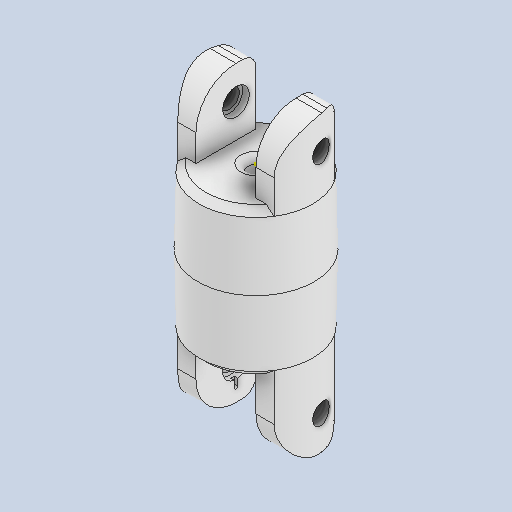
# Autodesk Inventor part: Index_1
Saved by Autodesk Inventor 2022 (Build 260153000, 153)
## iProperties
Created: 2023-01-15
Part Number: Index_1
Material: ABS Plastic
Document SubType Name: Modeling
Designer: 48735
Density: 1.06 g/cm^3
Appearance: Smooth - White
Author: 48735
Autodesk Inventor part; units mm, degrees
ref_plane "YZ Plane" through (0, 0, 0) normal (1, 0, 0) x (0, 1, 0)
ref_plane "XZ Plane" through (0, 0, 0) normal (0, 1, 0) x (-1, 0, 0)
ref_plane "XY Plane" through (0, 0, 0) normal (0, 0, 1) x (1, 0, 0)
sketch "Sketch1" plane through (0, 0, 0) normal (0, 1, 0) x (-1, 0, 0)
  line L0 (4.5, 0) -> (4.5, -4)
  line L1 (4.5, 0) -> (4.5, 4)
  line L2 (-4.5, 0) -> (-4.5, -4)
  line L3 (-4.5, 0) -> (-4.5, 4)
  circle A0 centre (0, 0) radius 8.5
  line L4 (4.5, 4) -> (4.5, 4.5)
  line L5 (-4.5, 4) -> (-4.5, 4.5)
  line L6 (-4.5, -4) -> (-4.5, -4.5)
  line L7 (-4.5, -4.5) -> (-7.2111, -4.5)
  line L8 (4.5, -4) -> (4.5, -4.5)
  line L9 (4.5, -4.5) -> (7.2111, -4.5)
  line L10 (4.5, 4) -> (4.5, 4.5)
  line L11 (4.5, 4.5) -> (7.2111, 4.5)
  line L12 (-4.5, 4) -> (-4.5, 4.5)
  line L13 (-4.5, 4.5) -> (-7.2111, 4.5)
  point P0 (7.5, 4)
  point P1 (7.5, -4)
  point P2 (-7.5, -4)
  point P3 (-7.5, 4)
  constraints: 28 end point, 3 point on line, 2 parallel, 2 perpendicular, 2 vertical, 1 coincident, 10 other
extrude "Extrusion1" add sketch "Sketch1" along normal blind 12 contours L1 L4 L11 A0 L9 L8 L0 | A0 L13 L5 L3 L2 L6 L7
sketch "Sketch2" plane through (0, 12, 0) normal (0, 1, 0) x (1, 0, 0)
  circle A0 centre (0, 0) radius 8.5
  circle A1 centre (0, 0) radius 1.25
  dimension "d11" = 17
  dimension "d12" = 2.5
  constraints: 2 centre point, 2 coincident
  measures "d11" diameter of A0
  measures "d12" diameter of A1
extrude "Extrusion2" add sketch "Sketch2" along normal blind 1
fillet "Fillet4" radius 6 2 edges at (-5.8556, 0, 4.5) (5.8556, 0, 4.5)
fillet "Fillet5" radius 2 2 edges at (5.8556, 0, -4.5) (-5.8556, 0, -4.5)
sketch "Sketch4" plane through (4.5, 12, -4.5) normal (-1, 0, 0) x (0, 0, 1)
  arc A0 (3, -12) -> (9, -6) centre (3, -6) ccw projected
  line L0 (3, -12) -> (3, -7)
  point P0 (4.5, -12)
  dimension "d30" = 5
  constraints: 2 end point, 1 vertical
  measures "d30" distance of L0.start L0.end
hole "Hole2" at (4.5, 5, -1.5) direction (1, 0, 0) diameter 3 depth 5 counterbore diameter 4 counterbore depth 1
sketch "Sketch5" plane through (-4.5, 12, 4.5) normal (1, 0, 0) x (0, 0, -1)
  line L0 (6, -12) -> (6, -7)
  point P0 (4.5, -12)
  dimension "d38" = 5
  constraints: 2 end point, 1 vertical
  measures "d38" distance of L0.start L0.end
hole "Hole3" at (-4.5, 5, -1.5) direction (-1, 0, 0) diameter 3 depth 5 counterbore diameter 4 counterbore depth 1
sketch "Sketch8" plane through (4.5, 12, -4.5) normal (-1, 0, 0) x (0, 0, 1)
  circle A0 centre (3, -7) radius 2 projected
  line L0 (3.25, -7) -> (3.25, -10)
  line L1 (2.75, -7) -> (2.75, -10)
  line L2 (3.25, -7) -> (2.75, -7)
  arc A1 (2.75, -10) -> (3.25, -10) centre (3, -10) ccw
  point P0 (4.5, -12)
  constraints: 6 end point, 2 point on circle, 1 centre point
extrude "Extrusion5" cut sketch "Sketch8" against normal blind 0.5 contours L1 L2 L0 A0 | A0 L0 A1 L1 picked at (2.9722, -7.6661)
sketch "Sketch9" plane through (5, 12, -4.5) normal (-1, 0, 0) x (0, 0, 1)
  arc A0 (2.75, -10) -> (3.25, -10) centre (3, -10) ccw projected
  circle A1 centre (3, -10) radius 0.25
  point P0 (4.5, -12)
  constraints: 1 centre point, 1 coincident
extrude "Extrusion6" cut sketch "Sketch9" against normal blind 0.5
sketch "Sketch10" plane through (-4.5, 12, 4.5) normal (1, 0, 0) x (0, 0, -1)
  circle A0 centre (6, -7) radius 2 projected
  line L0 (6.25, -7) -> (6.25, -10)
  line L1 (5.75, -7) -> (5.75, -10)
  line L2 (5.75, -7) -> (6.25, -7)
  arc A1 (5.75, -10) -> (6.25, -10) centre (6, -10) ccw
  point P0 (4.5, -12)
  constraints: 6 end point, 2 point on circle, 1 centre point
extrude "Extrusion7" cut sketch "Sketch10" against normal blind 0.5 contours L1 L2 L0 A0 | A0 L0 A1 L1 picked at (6.0278, -7.6661)
sketch "Sketch11" plane through (-5, 12, 4.5) normal (1, 0, 0) x (0, 0, -1)
  arc A0 (5.75, -10) -> (6.25, -10) centre (6, -10) ccw projected
  circle A1 centre (6, -10) radius 0.25
  point P0 (4.5, -12)
  constraints: 1 centre point, 1 coincident
extrude "Extrusion8" cut sketch "Sketch11" against normal blind 0.5
chamfer "Chamfer3" distance 1 angle 45 2 edges at (0, 12, 8.5) (0, 12, -8.5)
fillet "Fillet6" radius 1 1 edges at (-1.25, 12, 0)
sketch "Sketch12" plane through (0, 13, 0) normal (0, 1, 0) x (1, 0, 0)
  circle A0 centre (0, 0) radius 1.25
  circle A1 centre (0, 0) radius 8.7
  dimension "d79" = 17.4
  constraints: 2 centre point, 2 coincident
  measures "d79" diameter of A1
extrude "Extrusion9" add sketch "Sketch12" along normal blind 10
chamfer "Chamfer4" distance 10 distance2 0.2 1 edges at (-8.7, 13, 0) measured on face at (8.5873, 19.6667, 1.3956)
sketch "Sketch13" plane through (0, 23, 0) normal (0, 1, 0) x (1, 0, 0)
  circle A0 centre (0, 0) radius 1.25
  circle A1 centre (0, 0) radius 8.7
  dimension "d83" = 17.4
  constraints: 2 centre point, 2 coincident
  measures "d83" diameter of A1
extrude "Extrusion10" add sketch "Sketch13" along normal blind 10
chamfer "Chamfer5" distance 0.2 distance2 10 1 edges at (-8.7, 33, 0) measured on face at (6.1324, 33, 0.694)
sketch "Sketch14" plane through (0, 33, 0) normal (0, 1, 0) x (1, 0, 0)
  circle A0 centre (0, 0) radius 8.5
  circle A1 centre (0, 0) radius 1.25
  dimension "d91" = 17
  dimension "d90" = 2.5
  constraints: 2 centre point, 2 coincident
  measures "d91" diameter of A0
  measures "d90" diameter of A1
extrude "Extrusion11" add sketch "Sketch14" along normal blind 1
fillet "Fillet7" radius 1 1 edges at (-1.25, 34, 0)
sketch "Sketch15" plane through (0, 34, 0) normal (0, 1, 0) x (1, 0, 0)
  point P0 (0, 0)
sketch "Sketch16" plane through (0, 34, 0) normal (0, 1, 0) x (1, 0, 0)
  circle A0 centre (0, 0) radius 2.25 projected
  circle A1 centre (0, 0) radius 8.5
  circle A2 centre (0, 0) radius 1.25 projected
  line L0 (4.5, 0) -> (4.5, 4.5)
  line L1 (4.5, 4.5) -> (7.2111, 4.5)
  line L2 (4.5, -4.5) -> (4.5, 1.5) projected
  line L3 (4.5, 0) -> (4.5, -4.5)
  line L4 (7.2111, -4.5) -> (4.5, -4.5) projected
  line L5 (4.5, -4.5) -> (7.2111, -4.5)
  line L6 (-7.2111, 4.5) -> (-4.5, 4.5) projected
  line L7 (-4.5, 0) -> (-4.5, 4.5)
  line L8 (-4.5, 4.5) -> (-7.2111, 4.5)
  line L9 (-4.5, 0) -> (-4.5, -4.5)
  line L10 (-4.5, 1.5) -> (-4.5, -4.5) projected
  line L11 (-4.5, -4.5) -> (-7.2111, -4.5)
  point P0 (-7.2111, -4.5)
  point P1 (-7.2111, -4.5)
  constraints: 16 end point, 2 point on circle, 1 centre point, 1 coincident, 1 perpendicular, 1 vertical
extrude "Extrusion12" add sketch "Sketch16" along normal blind 10 contours A1 L4 L2 L0 L1 | L6 L7 L9 L11 A1
chamfer "Chamfer6" distance 1 angle 45 2 edges at (0, 34, 8.5) (0, 34, -8.5)
fillet "Fillet8" radius 6 2 edges at (-5.8556, 44, 4.5) (5.8556, 44, 4.5)
fillet "Fillet9" radius 2 2 edges at (5.8556, 44, -4.5) (-5.8556, 44, -4.5)
sketch "Sketch17" plane through (-4.5, 34, 4.5) normal (1, 0, 0) x (0, 0, -1)
  line L0 (6, 10) -> (7, 10) projected
  line L1 (6, 10) -> (6, 5)
  point P0 (4.5, -34)
  dimension "d106" = 5
  constraints: 2 end point, 1 vertical
  measures "d106" distance of L0.start L1.end
hole "Hole4" at (-4.5, 39, -1.5) direction (-1, 0, 0) diameter 3 depth 5 counterbore diameter 4 counterbore depth 1
sketch "Sketch18" plane through (4.5, 34, -4.5) normal (-1, 0, 0) x (0, 0, 1)
  arc A0 (9, 4) -> (3, 10) centre (3, 4) ccw projected
  line L0 (3, 10) -> (3, 5)
  point P0 (4.5, -34)
  dimension "d114" = 5
  constraints: 2 end point, 1 vertical
  measures "d114" distance of L0.start L0.end
hole "Hole5" at (4.5, 39, -1.5) direction (1, 0, 0) diameter 3 depth 5 counterbore diameter 4 counterbore depth 1
thread "Thread1" size "M3x0.5" class "6H" standard "ANSI Metric M Profile" length 6
thread "Thread2" size "M3x0.5" class "6H" standard "ANSI Metric M Profile" length 6
thread "Thread3" size "M3x0.5" class "6H" standard "ANSI Metric M Profile" length 6
thread "Thread4" size "M3x0.5" class "6H" standard "ANSI Metric M Profile" length 6
body "Solid1"
